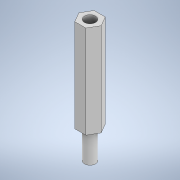
# Autodesk Inventor part: Spacer25mm
Saved by Autodesk Inventor 2022 (Build 260153000, 153)
## iProperties
Created: 2022-01-14
Part Number: Spacer25mm
Material: Generic
Document SubType Name: Modeling
Designer: Sergey
Density: 1 g/cm^3
Appearance: Default
Author: Sergey
Autodesk Inventor part; units mm, degrees
ref_plane "YZ Plane" through (0, 0, 0) normal (1, 0, 0) x (0, 1, 0)
ref_plane "XZ Plane" through (0, 0, 0) normal (0, 1, 0) x (-1, 0, 0)
ref_plane "XY Plane" through (0, 0, 0) normal (0, 0, 1) x (1, 0, 0)
sketch "Sketch1" plane through (0, 0, 0) normal (0, 1, 0) x (-1, 0, 0)
  line L0 (-3, 0) -> (-1.5, 2.5981)
  line L1 (-1.5, 2.5981) -> (1.5, 2.5981)
  line L2 (1.5, 2.5981) -> (3, 0)
  line L3 (3, 0) -> (1.5, -2.5981)
  line L4 (1.5, -2.5981) -> (-1.5, -2.5981)
  line L5 (-1.5, -2.5981) -> (-3, 0)
  point P0 (0, 0)
  point P1 (0, 0)
  dimension "d0" = 6
  constraints: 12 end point, 1 coincident, 1 horizontal alignment, 13 other
  measures "d0" distance of L0.start L2.end
sketch "Sketch2" plane through (0, 0, 0) normal (0, 1, 0) x (-1, 0, 0)
  point P0 (0, 0)
extrude "Extrusion1" add sketch "Sketch1" along normal blind 25
sketch "Sketch3" plane through (0, 0, 0) normal (0, -1, 0) x (1, 0, 0)
  circle A0 centre (0, 0) radius 1.5
  dimension "d3" = 3
  constraints: 1 centre point, 1 coincident
  measures "d3" diameter of A0
sketch "Sketch4" plane through (0, 25, 0) normal (0, 1, 0) x (1, 0, 0)
  circle A0 centre (0, 0) radius 1.5
  dimension "d4" = 3
  constraints: 1 centre point, 1 coincident
  measures "d4" diameter of A0
extrude "Extrusion2" add sketch "Sketch3" along normal blind 8
extrude "Extrusion3" cut sketch "Sketch4" against normal blind 10
body "Solid1"
